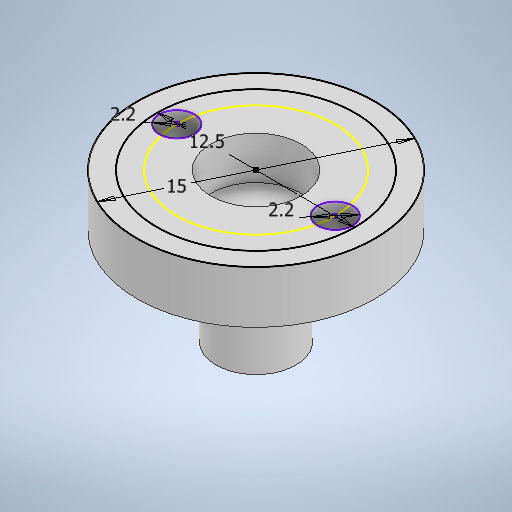
# Autodesk Inventor part: spinner_under
Saved by Autodesk Inventor 2025.2 (Build 292293000, 293)
## iProperties
Created: 2025-04-02
Part Number: spinner_under
Material: Generic
Document SubType Name: Modeling
Designer: m_kni
Density: 1 g/cm^3
Appearance: Default
Author: m_kni
## iProperties of the stored document spinner_under_3DPrint.ipt
Created: 2025-04-02
Part Number: spinner_under_3DPrint
Material: Generic
Document SubType Name: Modeling
Designer: m_kni
Density: 1 g/cm^3
Appearance: Default
Author: m_kni
Autodesk Inventor part; units mm, degrees
ref_plane "YZ Plane" through (0, 0, 0) normal (1, 0, 0) x (0, 1, 0)
ref_plane "XZ Plane" through (0, 0, 0) normal (0, 1, 0) x (-1, 0, 0)
ref_plane "XY Plane" through (0, 0, 0) normal (0, 0, 1) x (1, 0, 0)
sketch "Sketch1" plane through (0, 0, 0) normal (0, 1, 0) x (-1, 0, 0)
  circle A0 centre (0, 0) radius 2.525
  dimension "d0" = 5.05
  constraints: 1 centre point, 1 coincident
  measures "d0" diameter of A0
extrude "Extrusion1" add sketch "Sketch1" along normal blind 4
sketch "Sketch2" plane through (0, 4, 0) normal (0, 1, 0) x (1, 0, 0)
  circle A0 centre (0, 0) radius 5
  dimension "d3" = 10
  constraints: 1 centre point, 1 coincident
  measures "d3" diameter of A0
extrude "Extrusion2" add sketch "Sketch2" along normal blind 5.4
fillet "Fillet1" radius 2 1 edges at (-5, 4, 0)
sketch "Sketch3" plane through (0, 9.4, 0) normal (0, 1, 0) x (1, 0, 0)
  circle A0 centre (0, 0) radius 7.5
  circle A1 centre (0, 0) radius 6.25
  circle A2 centre (0, 0) radius 5 projected
  circle A3 centre (-5, 0) radius 1.1
  circle A4 centre (5, 0) radius 1.1
  point P0 (4.879, -1.0933)
  point P1 (-4.879, -1.0933)
  point P2 (-4.879, 1.0933)
  point P3 (4.879, 1.0933)
  dimension "d7" = 15
  dimension "d8" = 12.5
  dimension "d9" = 2.2
  dimension "d10" = 2.2
  constraints: 4 centre point, 2 coincident, 2 point on circle
  measures "d7" diameter of A0
  measures "d8" diameter of A1
  measures "d9" diameter of A3
  measures "d10" diameter of A4
extrude "Extrusion3" add sketch "Sketch3" against normal blind 3.3 contours A0 | A1
extrude "Extrusion4" cut sketch "Sketch3" against normal blind 5.4 contours A2 A4 | A2 A4 | A3 A2 | A2 A3
sketch "Sketch4" plane through (0, 6.1, 0) normal (0, -1, 0) x (1, 0, 0)
  arc A0 (4.879, -1.0933) -> (4.879, 1.0933) centre (5, 0) ccw projected
  arc A1 (-4.879, 1.0933) -> (-4.879, -1.0933) centre (-5, 0) ccw projected
  circle A2 centre (-5, 0) radius 2
  circle A3 centre (0, 0) radius 3 projected
  circle A4 centre (5, 0) radius 2
  constraints: 2 centre point, 2 coincident, 2 tangent
extrude "Extrusion5" cut sketch "Sketch4" along normal blind 3.3 contours A2 | A4
sketch "Sketch5" plane through (0, 0, 0) normal (1, 0, 0) x (0, 1, 0)
  point P0 (0, 0)
sketch "Sketch6" plane through (0, 9.4, 0) normal (0, 1, 0) x (1, 0, 0)
  circle A0 centre (0, 0) radius 2.85
  dimension "d17" = 5.7
  constraints: 1 centre point, 1 coincident
  measures "d17" diameter of A0
extrude "Extrusion6" cut sketch "Sketch6" against normal blind 2.7
body "Solid1"
